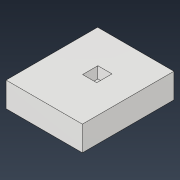
# Autodesk Inventor part: TCS3472
Saved by Autodesk Inventor 2022.1 (Build 261234020, 234B)
## iProperties
Part Number: TCS3472
Material: PC/ABS-Kunststoff
Document SubType Name: Modeling
Designer: rYan
Mass: 0.00109883 g
Surface Area: 0.15782 cm^2
Volume: 0.0030756 cm^3
Density: 0.357273 g/cm^3
Appearance: Glatt - Weiß
Author: rYan
Autodesk Inventor part; units mm, degrees
ref_plane "YZ Plane" through (0, 0, 0) normal (1, 0, 0) x (0, 1, 0)
ref_plane "XZ Plane" through (0, 0, 0) normal (0, 1, 0) x (-1, 0, 0)
ref_plane "XY Plane" through (0, 0, 0) normal (0, 0, 1) x (1, 0, 0)
sketch "Skizze1" plane through (0, 0, 0) normal (0, 0, 1) x (1, 0, 0)
  line L0 (-0.185, -0.2) -> (0.185, -0.2)
  line L1 (0.185, -0.2) -> (0.185, 0.2)
  line L2 (0.185, 0.2) -> (-0.185, 0.2)
  line L3 (-0.185, 0.2) -> (-0.185, -0.2)
  line L4 (-0.185, -0.2) -> (0.185, 0.2) construction
  line L5 (0.185, -0.2) -> (-0.185, 0.2) construction
  line L6 (-1.062, 1.071) -> (0.938, 1.071)
  line L7 (0.938, 1.071) -> (0.938, -1.329)
  line L8 (0.938, -1.329) -> (-1.062, -1.329)
  line L9 (-1.062, -1.329) -> (-1.062, 1.071)
  point P0 (0, 0)
  dimension "d0" = 0.37
  dimension "d1" = 0.4
  dimension "d2" = 0.877
  dimension "d3" = 0.871
  dimension "d4" = 2
  dimension "d5" = 2.4
  constraints: 20 end point, 4 parallel, 2 horizontal, 2 midpoint, 2 perpendicular
  measures "d0" distance of L1.end L2.end
  measures "d1" distance of L2.end L0.start
  measures "d2" distance between parallel lines of L9 L3
  measures "d3" distance between parallel lines of L6 L2
  measures "d4" distance of L6.start L6.end
  measures "d5" distance of L6.end L7.end
extrude "Extrusion1" add sketch "Skizze1" along normal blind 0.3
sketch "Skizze2" plane through (0, 0, 0) normal (0, 0, -1) x (-1, 0, 0)
  line L0 (0.185, 0.2) -> (0.185, -0.2) projected
  line L1 (0.185, -0.2) -> (-0.185, -0.2) projected
  line L2 (-0.185, -0.2) -> (-0.185, 0.2) projected
  line L3 (-0.185, 0.2) -> (0.185, 0.2) projected
  line L4 (1.062, 1.071) -> (-0.938, 1.071) projected
  line L5 (-0.938, 1.071) -> (-0.938, -1.329) projected
  line L6 (-0.938, -1.329) -> (1.062, -1.329) projected
  line L7 (1.062, -1.329) -> (1.062, 1.071) projected
  line L8 (-0.938, 1.071) -> (1.062, 1.071) projected
  line L9 (1.062, -1.329) -> (-0.938, -1.329)
  line L10 (-0.938, -1.329) -> (-0.938, 1.071)
  line L11 (-0.938, 1.071) -> (1.062, 1.071)
  line L12 (1.062, 1.071) -> (1.062, -1.329)
  point P0 (0, 0)
  constraints: 8 end point, 2 parallel, 1 horizontal, 1 perpendicular
extrude "Extrusion2" add sketch "Skizze2" along normal blind 0.35 contours L0 L1 L2 L3 | L7 L6 L5 L4
